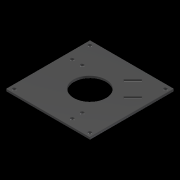
# Autodesk Inventor part: Bottom_Platform
Saved by Autodesk Inventor 2012 (Build 160160000, 160)
## iProperties
Created: 2012-10-03
Part Number: Bottom_Platform
Material: Polycarbonate, Clear
Document SubType Name: Modeling
Designer: agmlego
Density: 1.2 g/cm^3
Mass: 31.2648 g
Surface Area: 191.549 cm^2
Volume: 26.054 cm^3
Author: agmlego
Autodesk Inventor part; units mm, degrees
ref_plane "YZ Plane" through (0, 0, 0) normal (1, 0, 0) x (0, 1, 0)
ref_plane "XZ Plane" through (0, 0, 0) normal (0, 1, 0) x (-1, 0, 0)
ref_plane "XY Plane" through (0, 0, 0) normal (0, 0, 1) x (1, 0, 0)
sketch "Sketch1" plane through (0, 0, 0) normal (0, 0, 1) x (1, 0, 0)
  line L0 (-50, 50) -> (50, 50)
  line L1 (50, 50) -> (50, -50)
  line L2 (50, -50) -> (-50, -50)
  line L3 (-50, -50) -> (-50, 50)
  point P0 (0, 0)
  dimension "d0" = 100
  dimension "d1" = 50
  dimension "d2" = 50
  constraints: 8 end point, 2 parallel, 2 perpendicular, 1 horizontal
  measures "d0" distance of L2.end L0.start
  measures "d1" distance from line of L0 point (0, 0)
  measures "d2" distance from line of point (0, 0) L3
extrude "Extrusion1" add sketch "Sketch1" along normal blind 3
hole "Hole1" at (-45, 45, 3) direction (0, 0, -1) diameter 3.4 end through all clearance for "Flat Head Machine Screw" size "M3" standard "Ansi Metric M Profile"
hole "Hole2" at (45, 45, 3) direction (0, 0, -1) diameter 3.4 end through all clearance for "Flat Head Machine Screw" size "M3" standard "Ansi Metric M Profile"
hole "Hole3" at (45, -45, 3) direction (0, 0, -1) diameter 3.4 end through all clearance for "Flat Head Machine Screw" size "M3" standard "Ansi Metric M Profile"
hole "Hole4" at (-45, -45, 3) direction (0, 0, -1) diameter 3.4 end through all clearance for "Flat Head Machine Screw" size "M3" standard "Ansi Metric M Profile"
sketch "Sketch2" plane through (0, 0, 3) normal (0, 0, 1) x (1, 0, 0)
  circle A0 centre (-45, -45) radius 1.7 projected
  circle A1 centre (45, 45) radius 1.7 projected
  line L0 (21.0541, 40.5703) -> (10.4475, 29.9636)
  line L1 (10.4475, 29.9636) -> (12.286, 28.1252)
  line L2 (12.286, 28.1252) -> (22.8926, 38.7318)
  line L3 (22.8926, 38.7318) -> (21.0541, 40.5703)
  line L4 (38.7318, 22.8926) -> (28.1252, 12.286)
  line L5 (28.1252, 12.286) -> (29.9636, 10.4475)
  line L6 (29.9636, 10.4475) -> (40.5703, 21.0541)
  line L7 (40.5703, 21.0541) -> (38.7318, 22.8926)
  line L8 (45, 45) -> (-45, -45) construction
  line L9 (22.8926, 38.7318) -> (38.7318, 22.8926) construction
  circle A2 centre (0, 0) radius 28.575 construction
  point P0 (30.8122, 30.8122)
  dimension "d41" = 22.4
  dimension "d42" = 2.6
  dimension "d43" = 15
  dimension "d44" = 28.575
  dimension "d45" = 57.15
  constraints: 20 end point, 4 equal length, 3 collinear, 3 parallel, 3 perpendicular, 2 point on line, 1 centre point, 1 coincident, 1 midpoint
  measures "d41" distance between parallel lines of L4 L2
  measures "d42" distance between parallel lines of L2 L0
  measures "d43" distance between parallel lines of L1 L3
  measures "d44" distance from line of point (0, 0) L1
  measures "d45" diameter of A2
extrude "Extrusion2" cut sketch "Sketch2" against normal through all contours L3 L2 L1 L0 | L7 L6 L5 L4
sketch "Sketch3" plane through (0, 0, 3) normal (0, 0, 1) x (1, 0, 0)
  circle A0 centre (0, 0) radius 19.05
  dimension "d48" = 38.1
  constraints: 1 centre point, 1 coincident
  measures "d48" diameter of A0
extrude "Extrusion3" cut sketch "Sketch3" against normal through all
sketch "Sketch4" plane through (0, 0, 3) normal (0, 0, 1) x (1, 0, 0)
  line L0 (50, 50) -> (50, -50) projected
  line L1 (-50, 50) -> (50, 50) projected
  line L2 (-50, -50) -> (-50, 50) projected
  line L3 (50, -50) -> (-50, -50) projected
  line L4 (-29.046, 20) -> (-50, 20) construction
  line L5 (20, -29.046) -> (20, -50) construction
  point P0 (-40.986, 20)
  point P1 (20, -40.986)
  dimension "d51" = 11.94
  dimension "d52" = 11.94
  dimension "d53" = 9.014
  dimension "d54" = 9.014
  dimension "d55" = 30
  dimension "d56" = 30
  constraints: 4 end point, 4 point on line, 2 perpendicular
  measures "d51" distance of L4.start point (-40.986, 20)
  measures "d52" distance of point (20, -40.986) L5.start
  measures "d53" distance from line of L2 point (-40.986, 20)
  measures "d54" distance from line of L3 point (20, -40.986)
  measures "d55" distance from line of L1 point (-40.986, 20)
  measures "d56" distance from line of L0 point (20, -40.986)
hole "Hole5" at (-40.986, 20, 3) at (-29.046, 20, 3) at (20, -40.986, 3) at (20, -29.046, 3) direction (0, 0, -1) diameter 3.4 end through all clearance for "Flat Head Machine Screw" size "M3" standard "Ansi Metric M Profile"
fillet "Fillet1" radius 0.5 46 edges at (15.7508, 35.267, 3) (15.7508, 35.267, 0) (21.9733, 39.651, 0) (21.9733, 39.651, 3) (17.5893, 33.4285, 0) (17.5893, 33.4285, 3) (11.3667, 29.0444, 0) (11.3667, 29.0444, 3) (39.651, 21.9733, 0) (39.651, 21.9733, 3) (33.4285, 17.5893, 3) (33.4285, 17.5893, 0) (29.0444, 11.3667, 0) (29.0444, 11.3667, 3) (35.267, 15.7508, 0) (35.267, 15.7508, 3) (0, 50, 3) (0, 50, 0) (50, 0, 0) (50, 0, 3) (50, 50, 1.5) (-50, 50, 1.5) (-50, 0, 0) (-50, 0, 3) (-50, -50, 1.5) (0, -50, 3) (0, -50, 0) (50, -50, 1.5) (45, -43.3, 3) (45, -43.3, 0) (45, 46.7, 0) (45, 46.7, 3) (-45, 46.7, 0) (-45, 46.7, 3) (20, -39.286, 0) (20, -27.346, 0) (-40.986, 21.7, 0) (-29.046, 21.7, 0) (20, -39.286, 3) (20, -27.346, 3) (-40.986, 21.7, 3) (-29.046, 21.7, 3) (-19.05, 0, 0) (-19.05, 0, 3) (-45, -43.3, 0) (-45, -43.3, 3)
equation "\"d1\" = 0.5 * d0"
equation "\"d2\" = d1"
equation "\"d44\" = 0.5 * d45"
equation "\"d52\" = d51"
equation "\"d54\" = d53"
equation "\"d56\" = d55"
body "Solid1"
